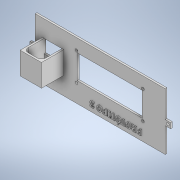
# Autodesk Inventor part: tampa
Saved by Autodesk Inventor 2022 (Build 260153000, 153)
## iProperties
Created: 2024-03-03
Part Number: tampa
Material: Genérico
Document SubType Name: Modeling
Designer: Daniel
Density: 1 g/cm^3
Appearance: Padrão
Author: Daniel
Autodesk Inventor part; units mm, degrees
ref_plane "YZ Plane" through (0, 0, 0) normal (1, 0, 0) x (0, 1, 0)
ref_plane "XZ Plane" through (0, 0, 0) normal (0, 1, 0) x (-1, 0, 0)
ref_plane "XY Plane" through (0, 0, 0) normal (0, 0, 1) x (1, 0, 0)
sketch "Esboço1" plane through (0, 0, 0) normal (0, 0, 1) x (1, 0, 0)
  line L0 (0, 0) -> (146, 0)
  line L1 (146, 0) -> (146, 64)
  line L2 (146, 64) -> (0, 64)
  line L3 (0, 64) -> (0, 0)
  dimension "d0" = 146
  dimension "d1" = 64
  constraints: 8 end point, 2 parallel, 1 horizontal, 1 perpendicular
  measures "d0" distance of L2.end L1.end
  measures "d1" distance of L1.end L0.end
extrude "Extrusão1" add sketch "Esboço1" along normal blind 2
sketch "Esboço2" plane through (0, 0, 2) normal (0, 0, 1) x (1, 0, 0)
  line L0 (0, 64) -> (0, 0) projected
  line L1 (0, 28) -> (-6, 28)
  line L2 (-6, 28) -> (-6, 34)
  line L3 (-6, 34) -> (0, 34)
  line L4 (0, 34) -> (0, 28)
  line L5 (146, 0) -> (146, 64) projected
  line L6 (146, 28) -> (152, 28)
  line L7 (152, 28) -> (152, 34)
  line L8 (152, 34) -> (146, 34)
  line L9 (146, 34) -> (146, 28)
  line L10 (146, 64) -> (0, 64) projected
  circle A0 centre (-3, 31) radius 1.5
  circle A1 centre (149, 31) radius 1.5
  point P0 (0, 34)
  dimension "d4" = 6
  dimension "d5" = 30
  dimension "d6" = 6
  dimension "d7" = 30
  dimension "d8" = 6
  dimension "d9" = 6
  dimension "d10" = 3
  dimension "d11" = 3
  dimension "d12" = 3
  dimension "d13" = 3
  dimension "d14" = 3
  dimension "d15" = 3
  constraints: 16 end point, 4 parallel, 2 centre point, 2 horizontal, 2 perpendicular, 2 point on line
  measures "d4" distance of L7.end L8.end
  measures "d5" distance from line of L5.end L8
  measures "d6" distance of L6.end L7.end
  measures "d7" distance between parallel lines of L10 L3
  measures "d8" distance of L1.end L2.end
  measures "d9" distance of L2.end L3.end
  measures "d10" diameter of A0
  measures "d11" diameter of A1
  measures "d12" distance from line of L8 A1.centre
  measures "d13" distance from line of L9 A1.centre
  measures "d14" distance from line of L0 A0.centre
  measures "d15" distance from line of L3 A0.centre
extrude "Extrusão2" add sketch "Esboço2" against normal blind 2
sketch "Esboço3" plane through (0, 0, 2) normal (0, 0, 1) x (1, 0, 0)
  circle A0 centre (46.483, 20) radius 1.5
  circle A1 centre (121, 20) radius 1.5
  circle A2 centre (46.483, 51.483) radius 1.5
  circle A3 centre (121, 51.483) radius 1.5
  line L0 (0, 64) -> (0, 34) projected
  line L1 (0, 0) -> (146, 0) projected
  line L2 (0, 28) -> (0, 0) projected
  line L3 (47.25, 49.5) -> (120.25, 49.5)
  line L4 (120.25, 49.5) -> (120.25, 22.5)
  line L5 (120.25, 22.5) -> (47.25, 22.5)
  line L6 (47.25, 22.5) -> (47.25, 49.5)
  line L7 (146, 34) -> (146, 64) projected
  line L8 (146, 0) -> (146, 28) projected
  dimension "d18" = 74.517
  dimension "d19" = 3
  dimension "d20" = 3
  dimension "d21" = 3
  dimension "d22" = 31.483
  dimension "d23" = 3
  dimension "d24" = 31.483
  dimension "d27" = 20
  dimension "d28" = 20
  dimension "d30" = 74.517
  dimension "d32" = 27
  dimension "d33" = 73
  dimension "d34" = 0.75
  dimension "d35" = 2.5
  dimension "d38" = 25
  dimension "d39" = 25
  constraints: 8 end point, 4 centre point, 2 parallel, 1 horizontal, 1 perpendicular
  measures "d18" distance of A0.centre A1.centre
  measures "d19" diameter of A0
  measures "d20" diameter of A1
  measures "d21" diameter of A2
  measures "d22" distance of A0.centre A2.centre
  measures "d23" diameter of A3
  measures "d24" distance of A1.centre A3.centre
  measures "d27" distance from line of L1 A1.centre
  measures "d28" distance from line of L1 A0.centre
  measures "d30" distance of A2.centre A3.centre
  measures "d32" distance of L3.end L4.end
  measures "d33" distance of L3.start L3.end
  measures "d34" distance from line of L4 A1.centre
  measures "d35" distance from line of A1.centre L5
  measures "d38" distance from line of L7 A3.centre
  measures "d39" distance from line of L8 A1.centre
extrude "Extrusão3" cut sketch "Esboço3" against normal blind 2
sketch "Esboço4" plane through (0, 0, 2) normal (0, 0, 1) x (1, 0, 0)
  point P0 (0, 0)
sketch "Esboço5" plane through (0, 0, 2) normal (0, 0, 1) x (1, 0, 0)
  point P0 (0, 0)
sketch "Esboço6" plane through (0, 0, 2) normal (0, 0, 1) x (1, 0, 0)
  line L0 (120.2026, 2.9574) -> (51.2957, 2.9574) construction
  line L1 (51.2957, 2.9574) -> (51.2957, 17.5984) construction
  line L2 (51.2957, 17.5984) -> (120.2026, 17.5984) construction
  line L3 (120.2026, 17.5984) -> (120.2026, 2.9574) construction
  line L4 (0, 0) -> (146, 0) projected
  line L5 (146, 0) -> (146, 28) projected
  spline S0 degree 2 poles (114.8787, 7.174) (114.8787, 7.5991) (115.1506, 8.3703) (115.4027, 8.6273) knots 0 0 0 1 2 2 2
  spline S1 degree 2 poles (115.4027, 8.6273) (115.5559, 8.7904) (115.9316, 9.0574) (116.154, 9.1513) knots 0 0 0 1 2 2 2
  spline S2 degree 2 poles (116.154, 9.1513) (116.3814, 9.2452) (116.9104, 9.354) (117.2366, 9.354) knots 0 0 0 1 2 2 2
  line L6 (117.2366, 9.354) -> (118.0374, 9.354)
  line L7 (118.0374, 9.354) -> (118.0374, 11.351)
  line L8 (118.0374, 11.351) -> (119.5699, 11.351)
  line L9 (119.5699, 11.351) -> (119.5699, 5.251)
  line L10 (119.5699, 5.251) -> (117.202, 5.251)
  spline S3 degree 2 poles (117.202, 5.251) (116.678, 5.251) (115.9118, 5.4438) (115.6004, 5.6515) knots 0 0 0 1 2 2 2
  spline S4 degree 2 poles (115.6004, 5.6515) (115.2544, 5.8838) (114.8787, 6.6451) (114.8787, 7.174) knots 0 0 0 1 2 2 2
  spline S5 degree 2 poles (116.4506, 7.2135) (116.4506, 6.9515) (116.6978, 6.5808) (116.8659, 6.5116) knots 0 0 0 1 2 2 2
  spline S6 degree 2 poles (116.8659, 6.5116) (117.0834, 6.4177) (117.4788, 6.388) (117.8199, 6.388) knots 0 0 0 1 2 2 2
  line L11 (117.8199, 6.388) -> (118.0374, 6.388)
  line L12 (118.0374, 6.388) -> (118.0374, 8.217)
  line L13 (118.0374, 8.217) -> (117.9287, 8.217)
  spline S7 degree 2 poles (117.9287, 8.217) (117.7161, 8.217) (117.3305, 8.2071) (117.1872, 8.1824) knots 0 0 0 1 2 2 2
  spline S8 degree 2 poles (117.1872, 8.1824) (117.0636, 8.1626) (116.7917, 8.044) (116.7176, 7.9699) knots 0 0 0 1 2 2 2
  spline S9 degree 2 poles (116.7176, 7.9699) (116.5594, 7.8216) (116.4506, 7.4904) (116.4506, 7.2135) knots 0 0 0 1 2 2 2
  line L14 (108.4228, 11.351) -> (110.2864, 11.351)
  line L15 (110.2864, 11.351) -> (111.9819, 9.1117)
  line L16 (111.9819, 9.1117) -> (112.5356, 9.1117)
  line L17 (112.5356, 9.1117) -> (112.5356, 11.351)
  line L18 (112.5356, 11.351) -> (114.0581, 11.351)
  line L19 (114.0581, 11.351) -> (114.0581, 5.251)
  line L20 (114.0581, 5.251) -> (111.6062, 5.251)
  spline S10 degree 2 poles (111.6062, 5.251) (111.0971, 5.251) (110.3457, 5.3796) (110.0244, 5.5773) knots 0 0 0 1 2 2 2
  spline S11 degree 2 poles (110.0244, 5.5773) (109.6981, 5.7849) (109.3126, 6.4325) (109.3126, 6.9268) knots 0 0 0 1 2 2 2
  spline S12 degree 2 poles (109.3126, 6.9268) (109.3126, 7.6238) (109.9453, 8.4988) (110.4742, 8.7558) knots 0 0 0 1 2 2 2
  line L21 (110.4742, 8.7558) -> (108.4228, 11.351)
  spline S13 degree 2 poles (110.8845, 7.1196) (110.8845, 6.8873) (111.0625, 6.5561) (111.2652, 6.4671) knots 0 0 0 1 2 2 2
  spline S14 degree 2 poles (111.2652, 6.4671) (111.4085, 6.4078) (111.7595, 6.3732) (112.0215, 6.3732) knots 0 0 0 1 2 2 2
  line L22 (112.0215, 6.3732) -> (112.5356, 6.3732)
  line L23 (112.5356, 6.3732) -> (112.5356, 8.0143)
  line L24 (112.5356, 8.0143) -> (112.0956, 8.0143)
  spline S15 degree 2 poles (112.0956, 8.0143) (111.7793, 8.0143) (111.3294, 7.9352) (111.1762, 7.8117) knots 0 0 0 1 2 2 2
  spline S16 degree 2 poles (111.1762, 7.8117) (111.0279, 7.693) (110.8845, 7.3767) (110.8845, 7.1196) knots 0 0 0 1 2 2 2
  spline S17 degree 2 poles (102.4167, 8.301) (102.4167, 9.784) (103.9985, 11.4796) (105.3728, 11.4796) knots 0 0 0 1 2 2 2
  spline S18 degree 2 poles (105.3728, 11.4796) (106.7519, 11.4796) (108.3239, 9.7643) (108.3239, 8.301) knots 0 0 0 1 2 2 2
  spline S19 degree 2 poles (108.3239, 8.301) (108.3239, 6.8329) (106.7519, 5.1225) (105.3728, 5.1225) knots 0 0 0 1 2 2 2
  spline S20 degree 2 poles (105.3728, 5.1225) (103.9985, 5.1225) (102.4167, 6.823) (102.4167, 8.301) knots 0 0 0 1 2 2 2
  spline S21 degree 2 poles (103.9985, 8.301) (103.9985, 7.7523) (104.221, 6.9861) (104.4138, 6.7439) knots 0 0 0 1 2 2 2
  spline S22 degree 2 poles (104.4138, 6.7439) (104.6066, 6.4918) (105.1009, 6.2743) (105.3678, 6.2743) knots 0 0 0 1 2 2 2
  spline S23 degree 2 poles (105.3678, 6.2743) (105.6496, 6.2743) (106.1093, 6.477) (106.3219, 6.734) knots 0 0 0 1 2 2 2
  spline S24 degree 2 poles (106.3219, 6.734) (106.5097, 6.9713) (106.7421, 7.7573) (106.7421, 8.301) knots 0 0 0 1 2 2 2
  spline S25 degree 2 poles (106.7421, 8.301) (106.7421, 8.8646) (106.5196, 9.6061) (106.3268, 9.8582) knots 0 0 0 1 2 2 2
  spline S26 degree 2 poles (106.3268, 9.8582) (106.134, 10.1103) (105.6348, 10.3278) (105.3678, 10.3278) knots 0 0 0 1 2 2 2
  spline S27 degree 2 poles (105.3678, 10.3278) (105.0959, 10.3278) (104.5917, 10.0955) (104.4088, 9.8483) knots 0 0 0 1 2 2 2
  spline S28 degree 2 poles (104.4088, 9.8483) (104.2111, 9.5814) (103.9985, 8.8745) (103.9985, 8.301) knots 0 0 0 1 2 2 2
  line L25 (100.3356, 11.351) -> (100.3356, 6.4127)
  line L26 (100.3356, 6.4127) -> (102.1399, 6.4127)
  line L27 (102.1399, 6.4127) -> (102.1399, 5.251)
  line L28 (102.1399, 5.251) -> (96.9989, 5.251)
  line L29 (96.9989, 5.251) -> (96.9989, 6.4127)
  line L30 (96.9989, 6.4127) -> (98.8032, 6.4127)
  line L31 (98.8032, 6.4127) -> (98.8032, 11.351)
  line L32 (98.8032, 11.351) -> (100.3356, 11.351)
  spline S29 degree 2 poles (90.8198, 8.301) (90.8198, 9.784) (92.4016, 11.4796) (93.7758, 11.4796) knots 0 0 0 1 2 2 2
  spline S30 degree 2 poles (93.7758, 11.4796) (95.155, 11.4796) (96.727, 9.7643) (96.727, 8.301) knots 0 0 0 1 2 2 2
  spline S31 degree 2 poles (96.727, 8.301) (96.727, 6.8329) (95.155, 5.1225) (93.7758, 5.1225) knots 0 0 0 1 2 2 2
  spline S32 degree 2 poles (93.7758, 5.1225) (92.4016, 5.1225) (90.8198, 6.823) (90.8198, 8.301) knots 0 0 0 1 2 2 2
  spline S33 degree 2 poles (92.4016, 8.301) (92.4016, 7.7523) (92.6241, 6.9861) (92.8169, 6.7439) knots 0 0 0 1 2 2 2
  spline S34 degree 2 poles (92.8169, 6.7439) (93.0096, 6.4918) (93.504, 6.2743) (93.7709, 6.2743) knots 0 0 0 1 2 2 2
  spline S35 degree 2 poles (93.7709, 6.2743) (94.0527, 6.2743) (94.5124, 6.477) (94.725, 6.734) knots 0 0 0 1 2 2 2
  spline S36 degree 2 poles (94.725, 6.734) (94.9128, 6.9713) (95.1451, 7.7573) (95.1451, 8.301) knots 0 0 0 1 2 2 2
  spline S37 degree 2 poles (95.1451, 8.301) (95.1451, 8.8646) (94.9227, 9.6061) (94.7299, 9.8582) knots 0 0 0 1 2 2 2
  spline S38 degree 2 poles (94.7299, 9.8582) (94.5371, 10.1103) (94.0378, 10.3278) (93.7709, 10.3278) knots 0 0 0 1 2 2 2
  spline S39 degree 2 poles (93.7709, 10.3278) (93.499, 10.3278) (92.9948, 10.0955) (92.8119, 9.8483) knots 0 0 0 1 2 2 2
  spline S40 degree 2 poles (92.8119, 9.8483) (92.6142, 9.5814) (92.4016, 8.8745) (92.4016, 8.301) knots 0 0 0 1 2 2 2
  line L33 (92.5054, 2.9574) -> (93.7363, 4.5689)
  line L34 (93.7363, 4.5689) -> (94.7101, 4.5689)
  line L35 (94.7101, 4.5689) -> (93.8599, 2.9574)
  line L36 (93.8599, 2.9574) -> (92.5054, 2.9574)
  line L37 (88.7387, 11.351) -> (88.7387, 6.4127)
  line L38 (88.7387, 6.4127) -> (90.5429, 6.4127)
  line L39 (90.5429, 6.4127) -> (90.5429, 5.251)
  line L40 (90.5429, 5.251) -> (85.4019, 5.251)
  line L41 (85.4019, 5.251) -> (85.4019, 6.4127)
  line L42 (85.4019, 6.4127) -> (87.2062, 6.4127)
  line L43 (87.2062, 6.4127) -> (87.2062, 11.351)
  line L44 (87.2062, 11.351) -> (88.7387, 11.351)
  line L45 (81.739, 11.351) -> (85.0213, 11.351)
  line L46 (85.0213, 11.351) -> (85.0213, 10.2882)
  line L47 (85.0213, 10.2882) -> (84.1464, 10.2882)
  line L48 (84.1464, 10.2882) -> (84.1464, 6.3139)
  line L49 (84.1464, 6.3139) -> (85.0213, 6.3139)
  line L50 (85.0213, 6.3139) -> (85.0213, 5.251)
  line L51 (85.0213, 5.251) -> (81.739, 5.251)
  line L52 (81.739, 5.251) -> (81.739, 6.3139)
  line L53 (81.739, 6.3139) -> (82.6139, 6.3139)
  line L54 (82.6139, 6.3139) -> (82.6139, 10.2882)
  line L55 (82.6139, 10.2882) -> (81.739, 10.2882)
  line L56 (81.739, 10.2882) -> (81.739, 11.351)
  spline S41 degree 2 poles (76.0295, 7.174) (76.0295, 7.5991) (76.3014, 8.3703) (76.5535, 8.6273) knots 0 0 0 1 2 2 2
  spline S42 degree 2 poles (76.5535, 8.6273) (76.7067, 8.7904) (77.0824, 9.0574) (77.3049, 9.1513) knots 0 0 0 1 2 2 2
  spline S43 degree 2 poles (77.3049, 9.1513) (77.5323, 9.2452) (78.0612, 9.354) (78.3874, 9.354) knots 0 0 0 1 2 2 2
  line L57 (78.3874, 9.354) -> (79.1882, 9.354)
  line L58 (79.1882, 9.354) -> (79.1882, 11.351)
  line L59 (79.1882, 11.351) -> (80.7207, 11.351)
  line L60 (80.7207, 11.351) -> (80.7207, 5.251)
  line L61 (80.7207, 5.251) -> (78.3528, 5.251)
  spline S44 degree 2 poles (78.3528, 5.251) (77.8288, 5.251) (77.0626, 5.4438) (76.7512, 5.6515) knots 0 0 0 1 2 2 2
  spline S45 degree 2 poles (76.7512, 5.6515) (76.4052, 5.8838) (76.0295, 6.6451) (76.0295, 7.174) knots 0 0 0 1 2 2 2
  spline S46 degree 2 poles (77.6015, 7.2135) (77.6015, 6.9515) (77.8486, 6.5808) (78.0167, 6.5116) knots 0 0 0 1 2 2 2
  spline S47 degree 2 poles (78.0167, 6.5116) (78.2342, 6.4177) (78.6297, 6.388) (78.9707, 6.388) knots 0 0 0 1 2 2 2
  line L62 (78.9707, 6.388) -> (79.1882, 6.388)
  line L63 (79.1882, 6.388) -> (79.1882, 8.217)
  line L64 (79.1882, 8.217) -> (79.0795, 8.217)
  spline S48 degree 2 poles (79.0795, 8.217) (78.8669, 8.217) (78.4814, 8.2071) (78.338, 8.1824) knots 0 0 0 1 2 2 2
  spline S49 degree 2 poles (78.338, 8.1824) (78.2144, 8.1626) (77.9425, 8.044) (77.8684, 7.9699) knots 0 0 0 1 2 2 2
  spline S50 degree 2 poles (77.8684, 7.9699) (77.7102, 7.8216) (77.6015, 7.4904) (77.6015, 7.2135) knots 0 0 0 1 2 2 2
  spline S51 degree 2 poles (69.6576, 8.301) (69.6576, 9.784) (71.2395, 11.4796) (72.6137, 11.4796) knots 0 0 0 1 2 2 2
  spline S52 degree 2 poles (72.6137, 11.4796) (73.9929, 11.4796) (75.5648, 9.7643) (75.5648, 8.301) knots 0 0 0 1 2 2 2
  spline S53 degree 2 poles (75.5648, 8.301) (75.5648, 6.8329) (73.9929, 5.1225) (72.6137, 5.1225) knots 0 0 0 1 2 2 2
  spline S54 degree 2 poles (72.6137, 5.1225) (71.2395, 5.1225) (69.6576, 6.823) (69.6576, 8.301) knots 0 0 0 1 2 2 2
  spline S55 degree 2 poles (71.2395, 8.301) (71.2395, 7.7523) (71.4619, 6.9861) (71.6547, 6.7439) knots 0 0 0 1 2 2 2
  spline S56 degree 2 poles (71.6547, 6.7439) (71.8475, 6.4918) (72.3418, 6.2743) (72.6087, 6.2743) knots 0 0 0 1 2 2 2
  spline S57 degree 2 poles (72.6087, 6.2743) (72.8905, 6.2743) (73.3502, 6.477) (73.5628, 6.734) knots 0 0 0 1 2 2 2
  spline S58 degree 2 poles (73.5628, 6.734) (73.7506, 6.9713) (73.983, 7.7573) (73.983, 8.301) knots 0 0 0 1 2 2 2
  spline S59 degree 2 poles (73.983, 8.301) (73.983, 8.8646) (73.7605, 9.6061) (73.5677, 9.8582) knots 0 0 0 1 2 2 2
  spline S60 degree 2 poles (73.5677, 9.8582) (73.375, 10.1103) (72.8757, 10.3278) (72.6087, 10.3278) knots 0 0 0 1 2 2 2
  spline S61 degree 2 poles (72.6087, 10.3278) (72.3369, 10.3278) (71.8327, 10.0955) (71.6498, 9.8483) knots 0 0 0 1 2 2 2
  spline S62 degree 2 poles (71.6498, 9.8483) (71.452, 9.5814) (71.2395, 8.8745) (71.2395, 8.301) knots 0 0 0 1 2 2 2
  spline S63 degree 2 poles (61.9758, 9.5023) (61.9758, 9.9521) (62.307, 10.6887) (62.6283, 10.9457) knots 0 0 0 1 2 2 2
  spline S64 degree 2 poles (62.6283, 10.9457) (62.9496, 11.2028) (63.8246, 11.4796) (64.4523, 11.4796) knots 0 0 0 1 2 2 2
  spline S65 degree 2 poles (64.4523, 11.4796) (65.1642, 11.4796) (66.1825, 11.2423) (66.5038, 11.094) knots 0 0 0 1 2 2 2
  line L65 (66.5038, 11.094) -> (66.5038, 9.7692)
  line L66 (66.5038, 9.7692) -> (66.3555, 9.7692)
  spline S66 degree 2 poles (66.3555, 9.7692) (66.0194, 9.9818) (65.1147, 10.2981) (64.7391, 10.2981) knots 0 0 0 1 2 2 2
  spline S67 degree 2 poles (64.7391, 10.2981) (64.5166, 10.2981) (63.9976, 10.219) (63.8196, 10.0905) knots 0 0 0 1 2 2 2
  spline S68 degree 2 poles (63.8196, 10.0905) (63.6812, 9.9867) (63.5131, 9.6852) (63.5131, 9.4133) knots 0 0 0 1 2 2 2
  spline S69 degree 2 poles (63.5131, 9.4133) (63.5131, 9.1414) (63.7504, 8.8498) (63.9481, 8.7805) knots 0 0 0 1 2 2 2
  spline S70 degree 2 poles (63.9481, 8.7805) (64.1459, 8.7113) (64.6946, 8.6965) (64.9071, 8.6965) knots 0 0 0 1 2 2 2
  line L67 (64.9071, 8.6965) -> (65.1691, 8.6965)
  line L68 (65.1691, 8.6965) -> (65.1691, 7.6238)
  line L69 (65.1691, 7.6238) -> (64.9269, 7.6238)
  spline S71 degree 2 poles (64.9269, 7.6238) (64.6501, 7.6238) (64.1805, 7.5744) (64.0173, 7.5002) knots 0 0 0 1 2 2 2
  spline S72 degree 2 poles (64.0173, 7.5002) (63.8542, 7.4211) (63.6713, 7.1443) (63.6713, 6.907) knots 0 0 0 1 2 2 2
  spline S73 degree 2 poles (63.6713, 6.907) (63.6713, 6.7192) (63.8443, 6.4869) (63.9679, 6.4226) knots 0 0 0 1 2 2 2
  spline S74 degree 2 poles (63.9679, 6.4226) (64.1162, 6.3485) (64.5117, 6.299) (64.6501, 6.299) knots 0 0 0 1 2 2 2
  spline S75 degree 2 poles (64.6501, 6.299) (64.8725, 6.299) (65.3421, 6.4028) (65.5596, 6.4869) knots 0 0 0 1 2 2 2
  spline S76 degree 2 poles (65.5596, 6.4869) (65.7327, 6.5511) (66.1083, 6.7587) (66.1973, 6.8131) knots 0 0 0 1 2 2 2
  line L70 (66.1973, 6.8131) -> (66.3258, 6.8131)
  line L71 (66.3258, 6.8131) -> (66.3258, 5.5081)
  spline S77 degree 2 poles (66.3258, 5.5081) (66.0095, 5.3746) (64.9417, 5.1225) (64.3831, 5.1225) knots 0 0 0 1 2 2 2
  spline S78 degree 2 poles (64.3831, 5.1225) (63.8394, 5.1225) (63.0386, 5.3104) (62.7568, 5.4933) knots 0 0 0 1 2 2 2
  spline S79 degree 2 poles (62.7568, 5.4933) (62.4454, 5.6861) (62.134, 6.2793) (62.134, 6.65) knots 0 0 0 1 2 2 2
  spline S80 degree 2 poles (62.134, 6.65) (62.134, 7.174) (62.737, 7.955) (63.2314, 8.0687) knots 0 0 0 1 2 2 2
  line L72 (63.2314, 8.0687) -> (63.2314, 8.128)
  spline S81 degree 2 poles (63.2314, 8.128) (63.0139, 8.1577) (62.5986, 8.3159) (62.4009, 8.4938) knots 0 0 0 1 2 2 2
  spline S82 degree 2 poles (62.4009, 8.4938) (62.218, 8.652) (61.9758, 9.1562) (61.9758, 9.5023) knots 0 0 0 1 2 2 2
  constraints: 2 other
extrude "Extrusão4" add sketch "Esboço6" along normal blind 1
sketch "Esboço8" plane through (0, 0, 2) normal (0, 0, 1) x (1, 0, 0)
  line L0 (30, 45) -> (10, 45)
  line L1 (10, 45) -> (10, 30)
  line L2 (10, 30) -> (30, 30)
  line L3 (30, 30) -> (30, 45)
  line L4 (0, 0) -> (146, 0) projected
  line L5 (0, 64) -> (0, 34) projected
  dimension "d50" = 20
  dimension "d51" = 15
  dimension "d52" = 30
  dimension "d53" = 10
  constraints: 8 end point, 2 parallel, 1 horizontal, 1 perpendicular
  measures "d50" distance of L2.end L1.end
  measures "d51" distance of L1.end L0.end
  measures "d52" distance between parallel lines of L4 L2
  measures "d53" distance between parallel lines of L5 L1
extrude "Extrusão6" cut sketch "Esboço8" against normal blind 10
sketch "Esboço9" plane through (0, 0, 2) normal (0, 0, 1) x (1, 0, 0)
  line L0 (10, 45) -> (30, 45) projected
  line L1 (30, 45) -> (32, 45)
  line L2 (32, 45) -> (32, 20)
  line L3 (32, 20) -> (30, 20)
  line L4 (30, 20) -> (30, 45)
  line L5 (30, 20) -> (10, 20)
  line L6 (10, 20) -> (10, 22)
  line L7 (10, 22) -> (30, 22)
  line L8 (30, 22) -> (30, 20)
  line L9 (10, 20) -> (8, 20)
  line L10 (8, 20) -> (8, 45)
  line L11 (8, 45) -> (10, 45)
  line L12 (10, 45) -> (10, 20)
  line L13 (10, 30) -> (10, 45) projected
  point P0 (0, 0)
  dimension "d56" = 2
  dimension "d57" = 25
  dimension "d58" = 2
  dimension "d59" = 0
  dimension "d60" = 2
  constraints: 24 end point, 6 parallel, 3 horizontal, 3 perpendicular, 1 point on line
  measures "d56" distance of L0.end L1.end
  measures "d57" distance of L1.end L2.end
  measures "d58" distance of L10.end L11.end
  measures "d59" distance between parallel lines of L13 L12
  measures "d60" distance between parallel lines of L5 L7
extrude "Extrusão7" add sketch "Esboço9" along normal blind 25 contours L12 L6 L9 L10 L11 | L1 L2 L3 L4 | L4 L5 L6 L7
sketch "Esboço10" plane through (0, 0, 27) normal (0, 0, 1) x (1, 0, 0)
  line L0 (30, 22) -> (30, 30) projected
  line L1 (10, 45) -> (10, 30) projected
  line L2 (30, 22) -> (10, 22)
  line L3 (10, 22) -> (10, 45)
  line L4 (10, 45) -> (30, 45)
  line L5 (30, 45) -> (30, 22)
  point P0 (0, 0)
  constraints: 8 end point, 2 parallel, 1 horizontal, 1 perpendicular
extrude "Extrusão8" add sketch "Esboço10" against normal blind 2
fillet "Arredondamento1" radius 5 3 edges at (10, 33.5, 25) (20, 22, 25) (30, 33.5, 25)
